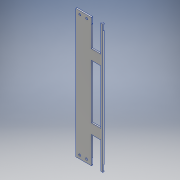
# Autodesk Inventor part: 앞뒷판_위_수정
Saved by Autodesk Inventor 2017 (Build 210142000, 142)
## iProperties
Part Number: 앞뒷판_위_수정
Material: 알루미늄 6061
Document SubType Name: Modeling
Designer: minom
Density: 2.7 g/cm^3
Appearance: 알루미늄 - 평지
Mass: 38.6128 g
Surface Area: 178.559 cm^2
Volume: 14.3011 cm^3
Author: minom
Autodesk Inventor part; units mm, degrees
ref_plane "YZ Plane" through (0, 0, 0) normal (1, 0, 0) x (0, 1, 0)
ref_plane "XZ Plane" through (0, 0, 0) normal (0, 1, 0) x (-1, 0, 0)
ref_plane "XY Plane" through (0, 0, 0) normal (0, 0, 1) x (1, 0, 0)
sketch "스케치1" plane through (0, 0, 0) normal (0, 1, 0) x (-1, 0, 0)
  line L0 (0, 0) -> (-40, 0)
  line L1 (-40, 0) -> (-40, -270)
  line L2 (-40, -270) -> (0, -270)
  line L3 (0, -270) -> (0, 0)
  dimension "d0" = 40
  dimension "d1" = 270
  constraints: 8 end point, 2 parallel, 1 horizontal, 1 perpendicular
  measures "d0" distance of L2.end L1.end
  measures "d1" distance of L1.end L0.end
extrude "돌출1" add sketch "스케치1" along normal blind 2
sketch "스케치2" plane through (0, 2, 0) normal (0, 1, 0) x (1, 0, 0)
  line L0 (0, 0) -> (40, 0) projected
  line L1 (40, 0) -> (40, 270) projected
  line L2 (40, 270) -> (0, 270) projected
  line L3 (0, 270) -> (0, 0) projected
  line L4 (0, 270) -> (0, 0) projected
  line L5 (40, 229) -> (0, 229)
  line L6 (0, 229) -> (0, 220.8)
  line L7 (0, 220.8) -> (40, 220.8)
  line L8 (40, 220.8) -> (40, 229)
  line L9 (40, 0) -> (40, 270) projected
  line L10 (40, 49.2) -> (0, 49.2)
  line L11 (0, 49.2) -> (0, 41)
  line L12 (0, 41) -> (40, 41)
  line L13 (40, 41) -> (40, 49.2)
  dimension "d4" = 8.2
  dimension "d5" = 8.2
  dimension "d6" = 41
  dimension "d7" = 41
  constraints: 16 end point, 4 parallel, 4 point on line, 2 horizontal, 2 perpendicular
  measures "d4" distance of L6.end L5.end
  measures "d5" distance of L11.end L10.end
  measures "d6" distance between parallel lines of L5 L2
  measures "d7" distance between parallel lines of L0 L12
extrude "돌출2" cut sketch "스케치2" against normal blind 1 contours L3 L10 L1 L12 | L3 L5 L1 L7
sketch "스케치3" plane through (0, 0, 0) normal (0, -1, 0) x (1, 0, 0)
  line L0 (0, 0) -> (40, 0) projected
  line L1 (0, -270) -> (0, 0) projected
  line L2 (40, -270) -> (0, -270) projected
  line L3 (40, 0) -> (40, -270) projected
  line L4 (37, -260) -> (37, -190)
  line L5 (37, -190) -> (23, -190)
  line L6 (23, -190) -> (23, -260)
  line L7 (23, -80) -> (37, -80)
  line L8 (37, -80) -> (37, -10)
  line L9 (37, -10) -> (23, -10)
  line L10 (23, -10) -> (23, -80)
  line L11 (23, -260) -> (37, -260)
  dimension "d15" = 14
  dimension "d17" = 3
  dimension "d20" = 14
  dimension "d21" = 70
  dimension "d22" = 3
  dimension "d23" = 10
  dimension "d25" = 10
  dimension "d26" = 70
  constraints: 16 end point, 3 parallel, 2 horizontal, 1 perpendicular
  measures "d15" distance of L5.end L4.end
  measures "d17" distance between parallel lines of L4 L3
  measures "d20" distance of L9.end L8.end
  measures "d21" distance of L8.end L7.end
  measures "d22" distance between parallel lines of L3 L8
  measures "d23" distance between parallel lines of L0 L9
  measures "d25" distance between parallel lines of L11 L2
  measures "d26" distance between parallel lines of L5 L11
extrude "돌출4" cut sketch "스케치3" against normal blind 2 contours L11 L6 L5 L4 | L10 L9 L8 L7
sketch "스케치4" plane through (0, 0, 0) normal (0, -1, 0) x (1, 0, 0)
  line L0 (23, -190) -> (37, -190) projected
  line L1 (37, -190) -> (37, -260) projected
  line L2 (37, -260) -> (23, -260) projected
  line L3 (23, -260) -> (23, -190) projected
  line L4 (37, -10) -> (37, -80) projected
  line L5 (37, -80) -> (23, -80) projected
  line L6 (23, -80) -> (23, -10) projected
  line L7 (23, -10) -> (37, -10) projected
  line L8 (0, 0) -> (40, 0) projected
  line L9 (0, -270) -> (0, 0) projected
  line L10 (40, -270) -> (0, -270) projected
  line L11 (40, 0) -> (40, -270) projected
  line L12 (23, -175) -> (37, -175)
  line L13 (37, -95) -> (23, -95)
  line L14 (23, -95) -> (23, -175)
  line L15 (37, -95) -> (37, -175)
  dimension "d36" = 95
  dimension "d39" = 14
  dimension "d40" = 3
  dimension "d41" = 80
  constraints: 8 end point, 1 horizontal, 1 parallel, 1 vertical
  measures "d36" distance between parallel lines of L8 L13
  measures "d39" distance between parallel lines of L15 L14
  measures "d40" distance between parallel lines of L11 L15
  measures "d41" distance between parallel lines of L12 L13
extrude "돌출6" cut sketch "스케치4" against normal blind 2 contours L14 L13 L15 L12
sketch "스케치5" plane through (0, 2, 0) normal (0, 1, 0) x (1, 0, 0)
  line L0 (40, 229) -> (40, 270) projected
  line L1 (0, 270) -> (0, 229) projected
  line L2 (40, 269) -> (0, 269)
  line L3 (0, 269) -> (0, 260.8)
  line L4 (0, 260.8) -> (40, 260.8)
  line L5 (40, 260.8) -> (40, 269)
  line L6 (40, 0) -> (40, 41) projected
  line L7 (0, 41) -> (0, 0) projected
  line L8 (40, 9.2) -> (0, 9.2)
  line L9 (0, 9.2) -> (0, 1)
  line L10 (0, 1) -> (40, 1)
  line L11 (40, 1) -> (40, 9.2)
  line L12 (0, 0) -> (40, 0) projected
  line L13 (40, 270) -> (0, 270) projected
  dimension "d44" = 8.2
  dimension "d45" = 8.2
  dimension "d46" = 1
  dimension "d47" = 1
  constraints: 16 end point, 4 parallel, 4 point on line, 2 horizontal, 2 perpendicular
  measures "d44" distance of L3.end L2.end
  measures "d45" distance of L9.end L8.end
  measures "d46" distance between parallel lines of L12 L10
  measures "d47" distance between parallel lines of L2 L13
extrude "돌출7" cut sketch "스케치5" against normal blind 1 contours L4 L1 L2 L0 | L10 L7 L8 L6
sketch "스케치6" plane through (0, 0, 0) normal (0, -1, 0) x (1, 0, 0)
  line L0 (0, -9.2) -> (40, -9.2) projected
  line L1 (40, -9.2) -> (40, -41) projected
  line L2 (40, -41) -> (37, -41) projected
  line L3 (37, -41) -> (37, -10) projected
  line L4 (37, -10) -> (23, -10) projected
  line L5 (23, -10) -> (23, -41) projected
  line L6 (23, -41) -> (0, -41) projected
  line L7 (0, -41) -> (0, -9.2) projected
  line L8 (37, -95) -> (23, -95) projected
  line L9 (23, -190) -> (23, -220.8) projected
  line L10 (23, -220.8) -> (0, -220.8) projected
  line L11 (0, -220.8) -> (0, -49.2) projected
  line L12 (0, -49.2) -> (23, -49.2) projected
  line L13 (23, -49.2) -> (23, -80) projected
  line L14 (23, -80) -> (37, -80) projected
  line L15 (37, -80) -> (37, -49.2) projected
  line L16 (37, -49.2) -> (40, -49.2) projected
  line L17 (40, -49.2) -> (40, -220.8) projected
  line L18 (40, -220.8) -> (37, -220.8) projected
  line L19 (37, -220.8) -> (37, -190) projected
  line L20 (40, -260.8) -> (0, -260.8) projected
  line L21 (0, -260.8) -> (0, -229) projected
  line L22 (0, -229) -> (23, -229) projected
  line L23 (23, -229) -> (23, -260) projected
  line L24 (23, -260) -> (37, -260) projected
  line L25 (37, -260) -> (37, -229) projected
  line L26 (37, -229) -> (40, -229) projected
  line L27 (40, -229) -> (40, -260.8) projected
  line L28 (0, -269) -> (40, -269) projected
  line L29 (40, -269) -> (40, -270) projected
  line L30 (40, -270) -> (0, -270) projected
  line L31 (0, -270) -> (0, -269) projected
  line L32 (40, -1) -> (0, -1) projected
  line L33 (0, -1) -> (0, 0) projected
  line L34 (0, 0) -> (40, 0) projected
  line L35 (40, 0) -> (40, -1) projected
  circle A0 centre (6, -5.1) radius 1.5
  circle A1 centre (16, -5.1) radius 1.5
  circle A2 centre (6, -45.1) radius 1.5
  circle A3 centre (16, -45.1) radius 1.5
  circle A4 centre (6, -224.9) radius 1.5
  circle A5 centre (16, -224.9) radius 1.5
  circle A6 centre (6, -264.9) radius 1.5
  circle A7 centre (16, -264.9) radius 1.5
  line L36 (0, -270) -> (0, 0) projected
  line L37 (37, -175) -> (37, -95) projected
  line L38 (23, -95) -> (23, -175) projected
  line L39 (23, -175) -> (37, -175) projected
  line L40 (37, -190) -> (23, -190) projected
  dimension "d50" = 3
  dimension "d51" = 3
  dimension "d52" = 3
  dimension "d53" = 3
  dimension "d54" = 3
  dimension "d55" = 3
  dimension "d56" = 3
  dimension "d57" = 3
  dimension "d58" = 4.1
  dimension "d59" = 6
  dimension "d60" = 4.1
  dimension "d61" = 10
  dimension "d62" = 4.1
  dimension "d63" = 4.1
  dimension "d64" = 6
  dimension "d65" = 10
  dimension "d66" = 4.1
  dimension "d67" = 4.1
  dimension "d68" = 6
  dimension "d69" = 10
  dimension "d70" = 4.1
  dimension "d71" = 4.1
  dimension "d72" = 6
  dimension "d73" = 10
  constraints: 8 centre point, 1 other
  measures "d50" diameter of A0
  measures "d51" diameter of A1
  measures "d52" diameter of A2
  measures "d53" diameter of A3
  measures "d54" diameter of A4
  measures "d55" diameter of A5
  measures "d56" diameter of A6
  measures "d57" diameter of A7
  measures "d58" distance from line of L0 A0.centre
  measures "d60" distance from line of L32 A1.centre
  measures "d61" distance of A0.centre A1.centre
  measures "d62" distance from line of L12 A2.centre
  measures "d63" distance from line of L6 A3.centre
  measures "d65" distance of A3.centre A2.centre
  measures "d66" distance from line of L22 A4.centre
  measures "d67" distance from line of L10 A5.centre
  measures "d69" distance of A5.centre A4.centre
  measures "d70" distance from line of L28 A6.centre
  measures "d71" distance from line of L20 A7.centre
  measures "d73" distance of A7.centre A6.centre
extrude "돌출8" cut sketch "스케치6" against normal blind 3 contours A0 | A1 | A2 | A3 | A4 | A5 | A6 | A7
sketch "스케치8" plane through (0, 2, 0) normal (0, 1, 0) x (1, 0, 0)
  line L0 (39, 40) -> (38, 40)
  line L1 (22, 40) -> (0, 40)
  line L2 (39, 230) -> (38, 230)
  line L3 (22, 230) -> (0, 230)
  line L4 (0, 40) -> (40, 40)
  line L5 (40, 40) -> (40, 0)
  line L6 (40, 0) -> (0, 0)
  line L7 (0, 0) -> (0, 40)
  line L8 (40, 270) -> (0, 270) projected
  line L9 (0, 230) -> (40, 230)
  line L10 (40, 230) -> (40, 270)
  line L11 (40, 270) -> (0, 270)
  line L12 (0, 270) -> (0, 230)
  constraints: 24 end point, 4 parallel, 2 horizontal, 2 perpendicular
extrude "돌출10" cut sketch "스케치8" against normal blind 2
